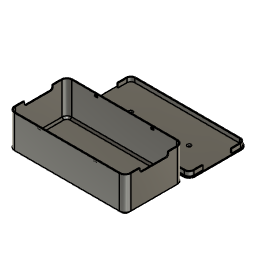
Cable Organizer V2 (Autodesk Fusion 360 design; units mm, degrees)
Autodesk Fusion 360 part; units mm, degrees
note: some values were not read from the file. Set by a fixed rule: which face or edge a step refers to.
sketch "Case Sketch" plane through (0, 0, 0) normal (0, 0, 1) x (1, 0, 0) in component "Case Closure"
  line L0 (0, 0) -> (200, 0)
  line L1 (200, 0) -> (200, 100)
  line L2 (200, 100) -> (0, 100)
  line L3 (0, 100) -> (0, 0)
  dimension "d1" = 200
  dimension "d2" = 100
  constraint horizontal L0
  constraint vertical L1
  constraint horizontal L2
  constraint vertical L3
  constraint coincident L0.start L3.end
  measures "d1" distance of L0.start L0.end
  measures "d2" distance of L0.start L2.end
extrude "Extrude1" add sketch "Case Sketch" along normal blind 60 makes body 1 in component "Case Closure"
fillet "Fillet1" radius 10 4 edges at (200, 0, 30) (200, 100, 30) (0, 0, 30) (0, 100, 30) on bodies 1 in component "Case Closure"
chamfer "Chamfer1" distance 4 angle 45 1 faces at (130, 33.3333, 0) on bodies 1 in component "Case Closure"
shell "Shell1" thickness 1.6 removed faces 1 at (130, 33.3333, 60) on bodies 1 in component "Case Closure"
sketch "Holes Sketch" plane through (0, 0, 0) normal (-1, 0, 0) x (0, -1, 0) in component "Case Closure"
  line L0 (-90, 4) -> (-10, 4)
  line L1 (-10, 4) -> (-10, 60)
  line L2 (-10, 60) -> (-90, 60)
  line L3 (-90, 60) -> (-90, 4)
  line L4 (-50, 60) -> (-50, 4) construction
  line L5 (-29, 53) -> (-71, 53)
  line L6 (-74.5, 56.5) -> (-74.5, 60)
  line L7 (-74.5, 60) -> (-25.5, 60)
  line L8 (-25.5, 60) -> (-25.5, 56.5)
  line L9 (-25.5, 53) -> (-74.5, 60) construction
  line L10 (-74.5, 53) -> (-25.5, 60) construction
  arc A0 (-74.5, 56.5) -> (-71, 53) centre (-71, 56.5) ccw
  arc A1 (-29, 53) -> (-25.5, 56.5) centre (-29, 56.5) ccw
  point P0 (-50, 56.5)
  dimension "d32" = 49
  dimension "d33" = 7
  dimension "d34" = 3.5
  dimension "d35" = 3.5
  constraint midpoint L2 L4.start
  constraint midpoint L0 L4.end
  constraint horizontal L5
  constraint perpendicular L5 L6
  constraint parallel L5 L7
  constraint parallel L6 L8
  constraint coincident L9 P0
  constraint coincident L10 P0
  constraint coincident L4 P0
  constraint coincident L4.start L7
  constraint coincident L10.start L5
  constraint coincident L10.start L6
  constraint tangent L5 A0
  constraint tangent L6 A0
  constraint coincident L9.start L5
  constraint coincident L9.start L8
  constraint tangent L5 A1
  constraint tangent L8 A1
  measures "d32" distance of L6.end L7.end
  measures "d33" distance of L10.start L6.end
  measures "d34" radius of A0
  measures "d35" radius of A1
extrude "Extrude2" cut sketch "Holes Sketch" against normal up to surface (1.6 mm away) contours L2 L5 L6 L7 L8 A0 A1 bodies 1 in component "Case Closure"
ref_plane "WorkPlane1" through (100, 50, 30) normal (-1, 0, 0) x (0, -1, 0) in component "Case Closure"
mirror "Mirror1" about plane through (100, 50, 30) normal (-1, 0, 0) of "Extrude2" in component "Case Closure"
sketch "Case Lid Sketch" plane through (0, 0, 0) normal (0, 0, 1) x (1, 0, 0) in component "Case Lid"
  line L0 (0, 0) -> (200, 0)
  line L1 (200, 0) -> (200, 100)
  line L2 (200, 100) -> (0, 100)
  line L3 (0, 100) -> (0, 0)
  dimension "d23" = 200
  dimension "d24" = 100
  constraint horizontal L0
  constraint vertical L1
  constraint horizontal L2
  constraint vertical L3
  constraint coincident L0.start L3.end
  measures "d23" distance of L0.start L0.end
  measures "d24" distance of L0.start L2.end
extrude "Extrude1'" add sketch "Case Lid Sketch" along normal blind 1.6 separate body makes body 2 in component "Case Lid"
fillet "Fillet1'" radius 10 4 edges at (200, 0, 0.8) (200, 100, 0.8) (0, 100, 0.8) (0, 0, 0.8) on bodies 2 in component "Case Lid"
sketch "Case Lid Edge Sketch" plane through (0, 0, 1.6) normal (0, 0, 1) x (-1, 0, 0) in component "Case Lid"
  arc A0 (0, -10) -> (-10, 0) centre (-10, -10) ccw
  line L0 (-10, 0) -> (-190, 0)
  arc A1 (-190, 0) -> (-200, -10) centre (-190, -10) ccw
  line L1 (-200, -10) -> (-200, -90)
  arc A2 (-200, -90) -> (-190, -100) centre (-190, -90) ccw
  line L2 (-190, -100) -> (-10, -100)
  arc A3 (-10, -100) -> (0, -90) centre (-10, -90) ccw
  line L3 (0, -90) -> (0, -10)
  line L4 (-10, -1.7) -> (-190, -1.7)
  arc A4 (-190, -1.7) -> (-198.3, -10) centre (-190, -10) ccw
  line L5 (-198.3, -10) -> (-198.3, -90)
  arc A5 (-198.3, -90) -> (-190, -98.3) centre (-190, -90) ccw
  line L6 (-190, -98.3) -> (-10, -98.3)
  arc A6 (-10, -98.3) -> (-1.7, -90) centre (-10, -90) ccw
  line L7 (-1.7, -90) -> (-1.7, -10)
  arc A7 (-1.7, -10) -> (-10, -1.7) centre (-10, -10) ccw
  line L8 (-10, -3.3) -> (-190, -3.3)
  arc A8 (-190, -3.3) -> (-196.7, -10) centre (-190, -10) ccw
  line L9 (-196.7, -10) -> (-196.7, -90)
  arc A9 (-196.7, -90) -> (-190, -96.7) centre (-190, -90) ccw
  line L10 (-190, -96.7) -> (-10, -96.7)
  arc A10 (-10, -96.7) -> (-3.3, -90) centre (-10, -90) ccw
  line L11 (-3.3, -90) -> (-3.3, -10)
  arc A11 (-3.3, -10) -> (-10, -3.3) centre (-10, -10) ccw
  dimension "d48" = -3.3
extrude "Extrude2'" add sketch "Case Lid Edge Sketch" along normal blind 7 contours L4 A4 L5 A5 L6 A6 L7 A7 bodies 2 in component "Case Lid"
sketch "Case Lid Holes Sketch" plane through (198.3, 0, 0) normal (1, 0, 0) x (0, 1, 0) in component "Case Lid"
  line L0 (10, 1.6) -> (90, 1.6)
  line L1 (90, 1.6) -> (90, 8.6)
  line L2 (90, 8.6) -> (10, 8.6)
  line L3 (10, 8.6) -> (10, 1.6)
  line L4 (50, 8.6) -> (50, 1.6) construction
  line L5 (74.5, 1.6) -> (25.5, 1.6)
  line L6 (25.5, 1.6) -> (25.5, 8.6)
  line L7 (25.5, 8.6) -> (74.5, 8.6)
  line L8 (74.5, 8.6) -> (74.5, 1.6)
  line L9 (74.5, 1.6) -> (25.5, 8.6) construction
  line L10 (25.5, 1.6) -> (74.5, 8.6) construction
  point P0 (50, 5.1)
  dimension "d49" = 49
  dimension "d50" = 7
  constraint midpoint L2 L4.start
  constraint midpoint L0 L4.end
  constraint horizontal L5
  constraint perpendicular L5 L6
  constraint parallel L5 L7
  constraint parallel L6 L8
  constraint coincident L9 P0
  constraint coincident L10 P0
  constraint midpoint L4 P0
  measures "d49" distance of L6.end L7.end
  measures "d50" distance of L5.end L6.end
extrude "Extrude4" cut sketch "Case Lid Holes Sketch" against normal up to surface (1.6 mm away) contours L0 L2 L5 L6 L7 L8 bodies 2 in component "Case Lid"
ref_plane "WorkPlane1" through (100, 50, 5.1) normal (1, 0, 0) x (0, 1, 0)
mirror "Mirror2" about plane through (100, 50, 5.1) normal (1, 0, 0) of "Extrude4" in component "Case Lid"
sketch "Case Lid Screw Holes Sketch" plane through (0, 0, 1.6) normal (0, 0, 1) x (-1, 0, 0) in component "Case Lid"
  line L0 (-1.7, -74.5) -> (-1.7, -90)
  arc A0 (-10, -98.3) -> (-1.7, -90) centre (-10, -90) ccw
  line L1 (-10, -98.3) -> (-190, -98.3)
  arc A1 (-198.3, -90) -> (-190, -98.3) centre (-190, -90) ccw
  line L2 (-198.3, -90) -> (-198.3, -74.5)
  line L3 (-198.3, -74.5) -> (-196.7, -74.5)
  line L4 (-196.7, -74.5) -> (-196.7, -90)
  line L5 (-190, -96.7) -> (-10, -96.7)
  line L6 (-3.3, -90) -> (-3.3, -74.5)
  line L7 (-3.3, -74.5) -> (-1.7, -74.5)
  arc A2 (0, -10) -> (-10, 0) centre (-10, -10) ccw
  line L8 (-10, 0) -> (-190, 0)
  arc A3 (-190, 0) -> (-200, -10) centre (-190, -10) ccw
  line L9 (-200, -10) -> (-200, -90)
  arc A4 (-200, -90) -> (-190, -100) centre (-190, -90) ccw
  line L10 (-190, -100) -> (-10, -100)
  arc A5 (-10, -100) -> (0, -90) centre (-10, -90) ccw
  line L11 (0, -90) -> (0, -10)
  line L12 (-1.7, -25.5) -> (-3.3, -25.5)
  line L13 (-3.3, -25.5) -> (-3.3, -10)
  line L14 (-10, -3.3) -> (-190, -3.3)
  line L15 (-196.7, -25.5) -> (-198.3, -25.5)
  line L16 (-198.3, -25.5) -> (-198.3, -10)
  arc A6 (-190, -1.7) -> (-198.3, -10) centre (-190, -10) ccw
  line L17 (-190, -1.7) -> (-10, -1.7)
  arc A7 (-1.7, -10) -> (-10, -1.7) centre (-10, -10) ccw
  line L18 (-1.7, -10) -> (-1.7, -25.5)
  circle A8 centre (-50, -50) radius 1.7
  circle A9 centre (-150, -50) radius 1.7
  arc A10 (-196.7, -90) -> (-190, -96.7) centre (-190, -90) ccw
  arc A11 (-10, -96.7) -> (-3.3, -90) centre (-10, -90) ccw
  arc A12 (-3.3, -10) -> (-10, -3.3) centre (-10, -10) ccw
  arc A13 (-190, -3.3) -> (-196.7, -10) centre (-190, -10) ccw
  line L19 (-196.7, -10) -> (-196.7, -25.5)
  line L20 (0, -50) -> (-200, -50) construction
  dimension "d56" = 3.4
  dimension "d57" = 50
  dimension "d60" = 3.4
  dimension "d61" = 50
  constraint midpoint L11 L20.start
  constraint midpoint L9 L20.end
  constraint coincident A9.centre L20
  constraint coincident A8.centre L20
  measures "d56" diameter of A8
  measures "d57" distance of L11 A8.centre
  measures "d60" diameter of A9
  measures "d61" distance of L9 A9.centre
extrude "Extrude5" cut sketch "Case Lid Screw Holes Sketch" against normal up to surface (1.6 mm away) contours A8 | A9 bodies 2 in component "Case Lid"
chamfer "Chamfer1'" distance 1.6 angle 45 2 edges at (151.585, 49.3853, 1.6) (51.585, 49.3853, 1.6) on bodies 2 in component "Case Lid"
sketch "Case Lid Peg Sketch" plane through (198.3, 0, 0) normal (1, 0, 0) x (0, 1, 0) in component "Case Lid"
  line L0 (74.5, 8.6) -> (74.5, 1.6)
  line L1 (74.5, 1.6) -> (90, 1.6)
  line L2 (90, 1.6) -> (90, 8.6)
  line L3 (90, 8.6) -> (74.5, 8.6)
  line L4 (98.3, 1.6) -> (98.3, 8.6) construction
  line L5 (98.3, 5.1) -> (99.1, 5.1) construction
  line L6 (99.1, 5.1) -> (98.3, 3.35)
  line L7 (99.1, 5.1) -> (98.3, 6.85)
  line L8 (98.3, 3.35) -> (98.3, 6.85)
  line L9 (99.1, 5.1) -> (99.2, 5.1) construction
  line L10 (99.2, 5.1) -> (98.3, 7.0687)
  line L11 (99.2, 5.1) -> (98.3, 3.1312)
  line L12 (98.3, 7.0687) -> (98.3, 6.85)
  line L13 (98.3, 3.1312) -> (98.3, 3.35)
  dimension "d65" = 0.8
  dimension "d66" = 1.75
  dimension "d67" = 0.1
  constraint midpoint L4 L5.start
  constraint perpendicular L4 L5
  constraint coincident L4 L6.end
  constraint coincident L4 L7.end
  constraint equal L6 L7
  constraint parallel L5 L9
  constraint coincident L4 L10.end
  constraint coincident L4 L11.end
  constraint parallel L6 L11
  constraint parallel L7 L10
  measures "d65" distance of L5.start L5.end
  measures "d66" distance of L5 L6.end
  measures "d67" distance of L5.end L9.end
extrude "Extrude6" add sketch "Case Lid Peg Sketch" along normal blind -47.5 and the other way blind 52.5 contours L6 L7 L8 bodies 2 in component "Case Lid"
mirror "Mirror3" about plane through (100, 50, 5.1) normal (1, 0, 0) of "Extrude6" in component "Case Lid"
ref_plane "WorkPlane2" through (100, 50, 5.1) normal (0, 1, 0) x (-1, 0, 0)
mirror "Mirror4" about plane through (100, 50, 5.1) normal (0, 1, 0) of "Extrude6", "Mirror3" in component "Case Lid"
ref_plane "WorkPlane3" through (100, 50, 30.8) normal (0, 0, 1) x (1, 0, 0)
mirror "Mirror5" about plane through (100, 50, 30.8) normal (0, 0, 1) of "Extrude6", "Mirror3", "Mirror4" makes body 3 at (149.1333, 98.3, 57.0833) makes body 4 at (50.8667, 98.3, 57.0833) makes body 5 at (149.1333, 1.7, 57.0833) makes body 6 at (50.8667, 1.7, 57.0833) in component "Case Lid"
combine "Combine1" operation cut target body 1 tool bodies 5 3 4 6 in component "Case Closure"
component "Case Closure" placed x (1, 0, 0) y (0, 1, 0) z (0, 0, 1) at (0, 0, 0)
component "Case Lid" placed x (1, 0, 0) y (0, 1, 0) z (0, 0, 1) at (0, 0, 0)
equation "d1 = CaseWidth"
equation "d2 = CaseDepth"
equation "d3 = CaseHeight"
equation "d6 = FilletSize"
equation "FilletSize = 10 mm"
equation "d8 = ChamferSize"
equation "ChamferSize = 4 mm"
equation "CaseThickness = 1.6 mm"
equation "d11 = CaseThickness"
equation "HolesSize = 7 mm"
equation "d23 = CaseWidth"
equation "d24 = CaseDepth"
equation "CaseWidth = 200 mm"
equation "CaseDepth = 100 mm"
equation "CaseHeight = 60 mm"
equation "d28 = CaseThickness"
equation "d31 = FilletSize"
equation "d32 = HolesSize * CablesCount"
equation "d33 = HolesSize"
equation "d34 = HolesSize / 2"
equation "d35 = HolesSize / 2"
equation "d38 = HolesSize"
equation "JoinTolerance = 0.1 mm"
equation "d47 = -CaseThickness - JoinTolerance"
equation "d48 = -JoinTolerance - CaseThickness * 2"
equation "d49 = HolesSize * CablesCount"
equation "d50 = HolesSize"
equation "CablesCount = 7"
equation "d56 = ScrewSize"
equation "d57 = CaseWidth / 4"
equation "ScrewSize = 3.4 mm"
equation "d60 = ScrewSize"
equation "d61 = CaseWidth / 4"
equation "d64 = CaseThickness"
equation "d65 = CaseThickness / 2"
equation "d66 = HolesSize / 4"
equation "d67 = JoinTolerance"
equation "d68 = -( CaseWidth / 4 - 2.5 mm )"
equation "d70 = CaseWidth / 4 + 2.5 mm"
equation "PegCount = 3"
